# Autodesk Inventor part: 1U
Saved by Autodesk Inventor 2016 SP1 (Build 200210100, 210)
## iProperties
Created: 2015-11-24
Part Number: 1U
Material: Generic
Document SubType Name: Modeling
Designer: PhillipD
Density: 1 g/cm^3
Appearance: CSMD0805, 1U
Author: PhillipD
Autodesk Inventor part; units mm, degrees
ref_plane "YZ Plane" through (0, 0, 0) normal (1, 0, 0) x (0, 1, 0)
ref_plane "XZ Plane" through (0, 0, 0) normal (0, 1, 0) x (-1, 0, 0)
ref_plane "XY Plane" through (0, 0, 0) normal (0, 0, 1) x (1, 0, 0)
sketch "CSMD0805, 1U_32" plane through (0, 0, 0) normal (0, 0, 1) x (1, 0, 0)
  line L0 (-0.9144, 0.6096) -> (0.9144, 0.6096)
  line L1 (0.9144, 0.6096) -> (0.9144, -0.6096)
  line L2 (0.9144, -0.6096) -> (-0.9144, -0.6096)
  line L3 (-0.9144, -0.6096) -> (-0.9144, 0.6096)
  constraints: 8 end point
extrude "Extrusion1" add sketch "CSMD0805, 1U_32" along normal blind 1
body "Solid1"
